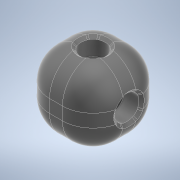
# Autodesk Inventor part: Nut
Saved by Autodesk Inventor 2022 (Build 260153000, 153)
## iProperties
Created: 2022-02-15
Part Number: Nut
Material: Generic
Document SubType Name: Modeling
Designer: Dahway
Density: 1 g/cm^3
Appearance: Smooth - Black
Author: Dahway
Autodesk Inventor part; units mm, degrees
ref_plane "YZ Plane" through (0, 0, 0) normal (1, 0, 0) x (0, 1, 0)
ref_plane "XZ Plane" through (0, 0, 0) normal (0, 1, 0) x (-1, 0, 0)
ref_plane "XY Plane" through (0, 0, 0) normal (0, 0, 1) x (1, 0, 0)
sketch "Sketch3" plane through (0, 0, 0) normal (0, 1, 0) x (-1, 0, 0)
  line L0 (0, -0.214) -> (12.1, -0.214)
  line L1 (12.1, -0.214) -> (12.1, -12.314)
  line L2 (12.1, -12.314) -> (0, -12.314)
  line L3 (0, -12.314) -> (0, -0.214)
  point P0 (0, 0)
  dimension "d6" = 12.1
  dimension "d7" = 12.1
  constraints: 8 end point, 2 parallel, 1 horizontal, 1 perpendicular
  measures "d6" distance of L1.end L2.end
  measures "d7" distance of L0.end L1.end
extrude "Extrusion2" add sketch "Sketch3" along normal blind 12.1
fillet "Fillet2" radius 5 12 edges at (0, 12.1, -6.264) (0, 6.05, -12.314) (-6.05, 12.1, -12.314) (-6.05, 12.1, -0.214) (-12.1, 12.1, -6.264) (-12.1, 6.05, -0.214) (0, 6.05, -0.214) (-12.1, 6.05, -12.314) (-6.05, 0, -12.314) (-12.1, 0, -6.264) (-6.05, 0, -0.214) (0, 0, -6.264)
sketch "Sketch4" plane through (0, 5, -7.314) normal (1, 0, 0) x (0, 0, -1)
  line L0 (0, 7.1) -> (-2.1, 7.1) projected
  line L1 (-7.1, 2.1) -> (-7.1, 0) projected
  point P0 (-7.314, -5)
  point P1 (-1.05, 1.05)
  dimension "d18" = 6.05
  dimension "d19" = 6.05
  measures "d18" distance from line of L0 point (-1.05, 1.05)
  measures "d19" distance from line of L1 point (-1.05, 1.05)
hole "Hole1" at (0, 6.05, -6.264) direction (-1, 0, 0) diameter 4 depth 3
sketch "Sketch5" plane through (-7.1, 5, -0.214) normal (0, 0, 1) x (1, 0, 0)
  line L0 (0, 0) -> (0, 2.1) projected
  line L1 (2.1, 0) -> (0, 0) projected
  point P0 (7.1, -5)
  point P1 (1.05, 1.05)
  dimension "d20" = 1.05
  dimension "d21" = 1.05
  measures "d20" distance from line of L0 point (1.05, 1.05)
  measures "d21" distance from line of L1 point (1.05, 1.05)
pattern_circular "Circular Pattern1" count 4 over 360 about axis through (-6.05, 6.05, -0.214) along (0, 0, 1) of "Hole1"
chamfer "Chamfer3" distance 0.5 angle 45 36 edges at (-4.6358, 0.0266, -4.8498) (-4.05, 0.0911, -6.264) (-4.6358, 0.0266, -7.6782) (-5.5123, 0.0774, -8.1904) (-6.5877, 0.0774, -8.1904) (-7.4642, 0.0266, -7.6782) (-8.05, 0.0911, -6.264) (-7.4642, 0.0266, -4.8498) (-6.05, 0.0911, -4.264) (-12.0734, 4.6358, -4.8498) (-12.0089, 4.05, -6.264) (-12.0734, 4.6358, -7.6782) (-12.0226, 5.5123, -8.1904) (-12.0226, 6.5877, -8.1904) (-12.0734, 7.4642, -7.6782) (-12.0089, 8.05, -6.264) (-12.0734, 7.4642, -4.8498) (-12.0089, 6.05, -4.264) (-7.4642, 12.0734, -4.8498) (-8.05, 12.0089, -6.264) (-7.4642, 12.0734, -7.6782) (-6.5877, 12.0226, -8.1904) (-5.5123, 12.0226, -8.1904) (-4.6358, 12.0734, -7.6783) (-4.05, 12.0089, -6.264) (-4.6358, 12.0734, -4.8498) (-6.05, 12.0089, -4.264) (-0.0266, 7.4642, -4.8498) (-0.0911, 8.05, -6.264) (-0.0266, 7.4642, -7.6782) (-0.0774, 6.5877, -8.1904) (-0.0774, 5.5123, -8.1904) (-0.0266, 4.6358, -7.6782) (-0.0911, 4.05, -6.264) (-0.0266, 4.6358, -4.8498) (-0.0911, 6.05, -4.264)
sketch "Sketch6" plane through (-5, 7.1, -12.314) normal (0, 0, -1) x (-1, 0, 0)
  line L0 (-5, 5) -> (7.1, 5)
  line L1 (7.1, 5) -> (7.1, -7.1)
  line L2 (7.1, -7.1) -> (-5, -7.1)
  line L3 (-5, -7.1) -> (-5, 5)
  dimension "d34" = 12.1
  dimension "d35" = 12.1
  constraints: 8 end point, 2 parallel, 1 horizontal, 1 perpendicular
  measures "d34" distance of L1.end L2.end
  measures "d35" distance of L0.end L1.end
extrude "Extrusion3" cut sketch "Sketch6" against normal blind 1
body "Solid2"
